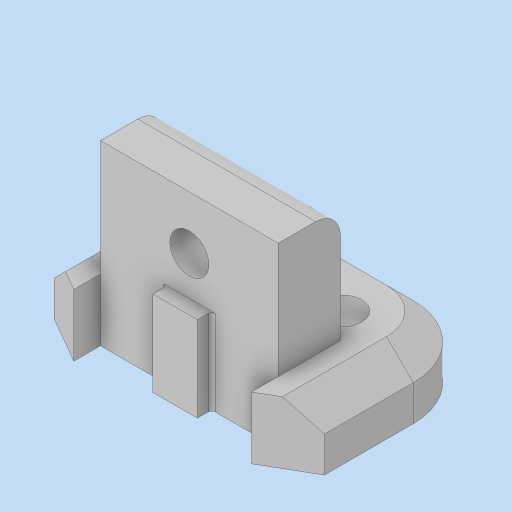
# Autodesk Inventor part: Ljoint
Saved by Autodesk Inventor 2024 (Build 280153000, 153)
## iProperties
Created: 2023-04-06
Part Number: Ljoint
Material: Generic
Document SubType Name: Modeling
Designer: Karbosch
Mass: 4.99579 g
Surface Area: 25.5982 cm^2
Volume: 4.99579 cm^3
Density: 1 g/cm^3
Appearance: Default
Author: Karbosch
Autodesk Inventor part; units mm, degrees
ref_plane "YZ Plane" through (0, 0, 0) normal (1, 0, 0) x (0, 1, 0)
ref_plane "XZ Plane" through (0, 0, 0) normal (0, 1, 0) x (-1, 0, 0)
ref_plane "XY Plane" through (0, 0, 0) normal (0, 0, 1) x (1, 0, 0)
sketch "Sketch1" plane through (0, 0, 0) normal (1, 0, 0) x (0, 1, 0)
  line L0 (0, 0) -> (20, 0)
  line L1 (20, 0) -> (20, -7)
  line L2 (20, -7) -> (0, -7)
  line L3 (0, -7) -> (0, 0)
  dimension "d18" = 20
  dimension "d19" = 7
  constraints: 8 end point, 2 parallel, 1 horizontal, 1 perpendicular
  measures "d18" distance of L1.end L2.end
  measures "d19" distance of L0.end L1.end
extrude "Extrusion1" add sketch "Sketch1" along normal blind 20
sketch "Sketch2" plane through (0, 8.5, -7) normal (0, 0, -1) x (-1, 0, 0)
  line L0 (0, 11.5) -> (0, 0) projected
  line L1 (0, 11.5) -> (-20, 11.5) projected
  line L2 (-20, 0) -> (-20, 11.5) projected
  line L3 (0, 0) -> (-20, 0) projected
  line L4 (0, 11.5) -> (-20, 11.5) projected
  line L5 (-10, 11.5) -> (-10, 5.5)
  circle A0 centre (-10, 5.5) radius 2.2
  line L6 (0, 11.5) -> (-20, 11.5) projected
  point P0 (0, -8.5)
  dimension "d6" = 6
  dimension "d7" = 4.4
  constraints: 2 end point, 1 centre point, 1 coincident, 1 midpoint, 1 perpendicular, 1 vertical
  measures "d6" distance of L5.start L5.end
  measures "d7" diameter of A0
extrude "Extrusion2" cut sketch "Sketch2" against normal through all contours A0
sketch "Sketch11" plane through (0, 0, -7) normal (0, -1, 0) x (1, 0, 0)
  line L0 (0, 0) -> (20, 0) projected
  line L1 (10, 0) -> (17.2, 0)
  line L2 (20, 7) -> (20, 0) projected
  arc A0 (17.2, -11) -> (25.2, -3) centre (17.2, -3) ccw
  line L3 (10, 0) -> (10, -11)
  line L4 (17.2, -11) -> (10, -11)
  line L5 (25.2, 7) -> (25.2, -3)
  circle A1 centre (17.2, -3) radius 2.2
  line L6 (0, 7) -> (20, 7) projected
  line L7 (25.2, 7) -> (20, 7)
  line L8 (20, 7) -> (20, 10)
  line L9 (20, 10) -> (25.2, 7)
  line L10 (17.2, -3) -> (17.2, 7)
  point P0 (13.4, 7)
  dimension "d58" = 7.2
  dimension "d66" = 4.4
  dimension "d72" = 3
  dimension "d73" = 10
  dimension "d75" = 8
  constraints: 16 end point, 4 point on circle, 2 centre point, 2 horizontal, 2 perpendicular, 2 point on line, 2 tangent, 2 vertical, 1 midpoint, 1 vertical alignment
  measures "d58" distance of L1.start L1.end
  measures "d66" diameter of A1
  measures "d72" distance of L2.start L8.end
  measures "d73" distance of L10.start L10.end
  measures "d75" distance from line of L4 A0.centre
extrude "Extrusion10" add sketch "Sketch11" against normal blind 7 contours L0 L2 L7 L5 A0 L4 L3 | L8 L9 L7
sketch "Sketch14" plane through (0, 7, -7) normal (0, 1, 0) x (1, 0, 0)
  circle A0 centre (17.2, 3) radius 2.2 projected
  circle A1 centre (17.2, 3) radius 3.6
  point P0 (0, -7)
  dimension "d76" = 7.2
  constraints: 1 centre point, 1 coincident
  measures "d76" diameter of A1
extrude "Extrusion11" cut sketch "Sketch14" along normal through all
mirror "Mirror4" about plane through (10, 0, -18) normal (-1, 0, 0) of "Extrusion10", "Extrusion11"
fillet "Fillet3" radius 2.8 1 edges at (10, 20, -7)
chamfer "Chamfer1" distance 3 angle 45 5 edges at (10, 7, -18) (-2.8569, 7, -15.6569) (-5.2, 7, -5) (22.8569, 7, -15.6569) (25.2, 7, -5)
sketch "Sketch15" plane through (0, 20, 0) normal (0, 0, 1) x (1, 0, 0)
  circle A0 centre (10, -6) radius 2.2 projected
  line L0 (10, -6) -> (10, -10.4)
  line L1 (2.8, -20) -> (17.2, -20) projected
  line L2 (7.5, -10.4) -> (12.5, -10.4)
  line L3 (12.5, -10.4) -> (12.5, -20)
  line L4 (12.5, -20) -> (7.5, -20)
  line L5 (7.5, -20) -> (7.5, -10.4)
  point P0 (0, -20)
  dimension "d83" = 4.4
  dimension "d84" = 5
  constraints: 10 end point, 2 parallel, 1 horizontal, 1 midpoint, 1 perpendicular, 1 point on line, 1 vertical
  measures "d83" distance of L0.end L0.start
  measures "d84" distance of L3.end L4.end
extrude "Extrusion12" add sketch "Sketch15" along normal blind 1.6 contours L2 L3 L1 L5
fillet "Fillet4" radius 0.4 2 edges at (12.5, 4.8, 0) (7.5, 4.8, 0)
body "Solid1"
